Autodesk Inventor part; units mm, degrees
(part 2 of 2)
  spline S40 degree 3 poles (29.0897, 30.1625) (29.0266, 29.976) (28.9005, 29.603) (28.6866, 29.0523) (28.4534, 28.5096) (28.24, 28.066) (28.057, 27.7174) (27.9126, 27.4598) (27.7629, 27.2052) (27.6252, 27.0011) (27.525, 26.8315) (27.4755, 26.7183) (27.4493, 26.6233) (27.4363, 26.5506) (27.4305, 26.477) (27.4338, 26.403) (27.4493, 26.3306) (27.4734, 26.2607) (27.5066, 26.1943) (27.5982, 26.0779) (27.7581, 25.9243) (27.9005, 25.7542) (28.0104, 25.6549) (28.0744, 25.6173) (28.1424, 25.5885) (28.2136, 25.5681) (28.2872, 25.5597) (28.3611, 25.5605) (28.4345, 25.5685) (28.531, 25.5881) (28.6474, 25.6298) (28.8234, 25.7182) (29.0363, 25.8416) (29.3006, 25.9736) (29.5674, 26.1001) (29.9277, 26.2589) (30.3849, 26.4415) (30.9423, 26.6371) (31.5062, 26.8129) (31.8869, 26.9133) (32.0773, 26.9635) knots 0 0 0 0 0.059055 0.118109 0.177163 0.236216 0.265745 0.295273 0.3248 0.354329 0.36909 0.383846 0.391225 0.398597 0.405969 0.413352 0.420732 0.428104 0.435485 0.442861 0.472389 0.501917 0.509293 0.516674 0.524045 0.531426 0.538808 0.54618 0.553552 0.560931 0.575687 0.590449 0.619977 0.649505 0.679033 0.708561 0.767614 0.826668 0.885723 0.944777 0.944777 0.944777 0.944777
  spline S41 degree 3 poles (24.7117, 33.8426) (24.6746, 33.6492) (24.6004, 33.2625) (24.4634, 32.6879) (24.3064, 32.1185) (24.1553, 31.6499) (24.0215, 31.2796) (23.9135, 31.0048) (23.7999, 30.7321) (23.6913, 30.5112) (23.6151, 30.3296) (23.5814, 30.2107) (23.5685, 30.1131) (23.5655, 30.0393) (23.5698, 29.9655) (23.5831, 29.8926) (23.6083, 29.823) (23.6417, 29.7571) (23.6836, 29.6959) (23.7902, 29.593) (23.9695, 29.4625) (24.1338, 29.3135) (24.2562, 29.23) (24.3246, 29.2015) (24.396, 29.1822) (24.4693, 29.1717) (24.5433, 29.1734) (24.6164, 29.1842) (24.6881, 29.2022) (24.781, 29.2347) (24.8906, 29.2919) (25.0529, 29.4035) (25.2471, 29.5547) (25.491, 29.7214) (25.7381, 29.8831) (26.0734, 30.0894) (26.5014, 30.3327) (27.027, 30.6023) (27.5617, 30.8533) (27.9252, 31.0046) (28.107, 31.0803) knots 0 0 0 0 0.059055 0.118109 0.177163 0.236216 0.265745 0.295273 0.3248 0.354329 0.36909 0.383846 0.391225 0.398597 0.405969 0.413352 0.420732 0.428104 0.435485 0.442861 0.472389 0.501917 0.509293 0.516674 0.524045 0.531426 0.538808 0.54618 0.553552 0.560931 0.575687 0.590449 0.619977 0.649505 0.679033 0.708561 0.767614 0.826668 0.885723 0.944777 0.944777 0.944777 0.944777
  spline S42 degree 3 poles (19.8733, 36.8923) (19.8628, 36.6957) (19.842, 36.3025) (19.7846, 35.7145) (19.7065, 35.1291) (19.6207, 34.6443) (19.5385, 34.2592) (19.4689, 33.9723) (19.3935, 33.6866) (19.316, 33.453) (19.2653, 33.2627) (19.2481, 33.1403) (19.2486, 33.0418) (19.2556, 32.9683) (19.2699, 32.8958) (19.2931, 32.8255) (19.3275, 32.7599) (19.3696, 32.6991) (19.4194, 32.6442) (19.539, 32.5568) (19.7345, 32.452) (19.9175, 32.3267) (20.0501, 32.2607) (20.1218, 32.2417) (20.1951, 32.2323) (20.2692, 32.2319) (20.3423, 32.2437) (20.4132, 32.2643) (20.4818, 32.2919) (20.5694, 32.3368) (20.6702, 32.4084) (20.8158, 32.541) (20.9876, 32.7173) (21.2065, 32.9156) (21.4293, 33.1094) (21.7334, 33.3595) (22.1243, 33.6588) (22.6082, 33.9974) (23.1038, 34.3189) (23.4433, 34.5183) (23.6131, 34.618) knots 0 0 0 0 0.059055 0.118109 0.177163 0.236216 0.265745 0.295273 0.3248 0.354329 0.36909 0.383846 0.391225 0.398597 0.405969 0.413352 0.420732 0.428104 0.435485 0.442861 0.472389 0.501917 0.509293 0.516674 0.524045 0.531426 0.538808 0.54618 0.553552 0.560931 0.575687 0.590449 0.619977 0.649505 0.679033 0.708561 0.767614 0.826668 0.885723 0.944777 0.944777 0.944777 0.944777
  spline S43 degree 3 poles (14.6647, 39.2547) (14.6811, 39.0585) (14.714, 38.6662) (14.7372, 38.0759) (14.7395, 37.4852) (14.7205, 36.9933) (14.6916, 36.6006) (14.6617, 36.3069) (14.6259, 36.0136) (14.5809, 35.7716) (14.5566, 35.5762) (14.5562, 35.4526) (14.5701, 35.3551) (14.5871, 35.2832) (14.6111, 35.2134) (14.6436, 35.1468) (14.6867, 35.0865) (14.7366, 35.0321) (14.7935, 34.9844) (14.9239, 34.9141) (15.1318, 34.8369) (15.3301, 34.7377) (15.4705, 34.6904) (15.5442, 34.6813) (15.618, 34.682) (15.6915, 34.6916) (15.7623, 34.7133) (15.8298, 34.7434) (15.8939, 34.7801) (15.9747, 34.8365) (16.0647, 34.9211) (16.1909, 35.0723) (16.3371, 35.2703) (16.527, 35.4967) (16.7213, 35.719) (16.9885, 36.0082) (17.335, 36.3579) (17.7683, 36.7593) (18.2156, 37.1452) (18.5248, 37.389) (18.6793, 37.5109) knots 0 0 0 0 0.059055 0.118109 0.177163 0.236216 0.265745 0.295273 0.3248 0.354329 0.36909 0.383846 0.391225 0.398597 0.405969 0.413352 0.420732 0.428104 0.435485 0.442861 0.472389 0.501917 0.509293 0.516674 0.524045 0.531426 0.538808 0.54618 0.553552 0.560931 0.575687 0.590449 0.619977 0.649505 0.679033 0.708561 0.767614 0.826668 0.885723 0.944777 0.944777 0.944777 0.944777
  spline S44 degree 3 poles (9.1829, 40.8859) (9.2259, 40.6938) (9.3119, 40.3096) (9.4152, 39.728) (9.498, 39.1431) (9.5461, 38.6532) (9.571, 38.2602) (9.5814, 37.9651) (9.5858, 37.6698) (9.5742, 37.4239) (9.5767, 37.227) (9.5932, 37.1045) (9.6202, 37.0097) (9.6468, 36.9409) (9.6802, 36.8749) (9.7214, 36.8134) (9.7723, 36.7596) (9.8292, 36.7124) (9.892, 36.673) (10.0308, 36.6211) (10.2472, 36.5728) (10.4572, 36.5016) (10.6027, 36.4738) (10.6769, 36.4749) (10.75, 36.4856) (10.8215, 36.5052) (10.8887, 36.5363) (10.9514, 36.5753) (11.01, 36.6203) (11.0823, 36.6872) (11.16, 36.7833) (11.2645, 36.9503) (11.3823, 37.1664) (11.5396, 37.4165) (11.7018, 37.6632) (11.9272, 37.9861) (12.2229, 38.3797) (12.5975, 38.8363) (12.988, 39.2796) (13.2611, 39.5632) (13.3976, 39.705) knots 0 0 0 0 0.059055 0.118109 0.177163 0.236216 0.265745 0.295273 0.3248 0.354329 0.36909 0.383846 0.391225 0.398597 0.405969 0.413352 0.420732 0.428104 0.435485 0.442861 0.472389 0.501917 0.509293 0.516674 0.524045 0.531426 0.538808 0.54618 0.553552 0.560931 0.575687 0.590449 0.619977 0.649505 0.679033 0.708561 0.767614 0.826668 0.885723 0.944777 0.944777 0.944777 0.944777
  spline S45 degree 3 poles (3.5301, 41.7555) (3.5988, 41.5711) (3.7363, 41.2021) (3.9179, 40.64) (4.0796, 40.0719) (4.194, 39.593) (4.272, 39.2071) (4.3225, 38.9162) (4.3671, 38.6242) (4.3891, 38.379) (4.4184, 38.1842) (4.4514, 38.0651) (4.4911, 37.975) (4.5269, 37.9104) (4.5689, 37.8496) (4.6181, 37.7943) (4.6758, 37.7478) (4.7386, 37.7089) (4.8062, 37.6783) (4.9508, 37.6458) (5.1718, 37.6275) (5.3895, 37.5855) (5.5375, 37.5778) (5.6108, 37.589) (5.6818, 37.6096) (5.7499, 37.6387) (5.8123, 37.6787) (5.8691, 37.7259) (5.921, 37.7784) (5.9835, 37.8546) (6.0474, 37.9603) (6.1281, 38.14) (6.2155, 38.3701) (6.3372, 38.6393) (6.4643, 38.9058) (6.6436, 39.2563) (6.883, 39.6865) (7.1919, 40.19) (7.5184, 40.6823) (7.7504, 41.0004) (7.8664, 41.1595) knots 0 0 0 0 0.059055 0.118109 0.177163 0.236216 0.265745 0.295273 0.3248 0.354329 0.36909 0.383846 0.391225 0.398597 0.405969 0.413352 0.420732 0.428104 0.435485 0.442861 0.472389 0.501917 0.509293 0.516674 0.524045 0.531426 0.538808 0.54618 0.553552 0.560931 0.575687 0.590449 0.619977 0.649505 0.679033 0.708561 0.767614 0.826668 0.885723 0.944777 0.944777 0.944777 0.944777
  circle A4 centre (0, 0) radius 5
  circle A5 centre (0, 0) radius 10
  circle A6 centre (0, 0) radius 33
  line L0 (0, -58.6663) -> (0, 58.6663) construction
  line L1 (-5, 8.6603) -> (-5, 32.619)
  line L2 (5, 8.6603) -> (5, 32.619)
  line L3 (-8.6603, -5) -> (-32.619, -5)
  line L4 (-8.6603, 5) -> (-32.619, 5)
  line L5 (5, -8.6603) -> (5, -32.619)
  line L6 (-5, -8.6603) -> (-5, -32.619)
  line L7 (8.6603, 5) -> (32.619, 5)
  line L8 (8.6603, -5) -> (32.619, -5)
  point P0 (-1.9127, 41.3251)
  point P1 (-1.6555, 40.7935)
  point P2 (-1.4188, 40.2525)
  point P3 (-1.205, 39.702)
  point P4 (-1.1077, 39.4232)
  point P5 (-1.0178, 39.142)
  point P6 (-0.9358, 38.8583)
  point P7 (-0.8628, 38.5722)
  point P8 (-0.8193, 38.4311)
  point P9 (-0.7593, 38.2963)
  point P10 (-0.7207, 38.2334)
  point P11 (-0.6765, 38.1744)
  point P12 (-0.6265, 38.1203)
  point P13 (-0.57, 38.0727)
  point P14 (-0.507, 38.0343)
  point P15 (-0.4396, 38.0044)
  point P16 (-0.3686, 37.9843)
  point P17 (-0.2953, 37.9763)
  point P18 (0, 37.976)
  point P19 (0.2953, 37.9763)
  point P20 (0.3686, 37.9843)
  point P21 (0.4396, 38.0044)
  point P22 (0.507, 38.0343)
  point P23 (0.57, 38.0727)
  point P24 (0.6265, 38.1203)
  point P25 (0.6765, 38.1744)
  point P26 (0.7207, 38.2334)
  point P27 (0.7593, 38.2963)
  point P28 (0.8193, 38.4311)
  point P29 (0.8628, 38.5722)
  point P30 (0.9358, 38.8583)
  point P31 (1.0178, 39.142)
  point P32 (1.1077, 39.4232)
  point P33 (1.205, 39.702)
  point P34 (1.4188, 40.2525)
  point P35 (1.6555, 40.7935)
  point P36 (1.9127, 41.3251)
  point P37 (-7.522, 40.6798)
  point P38 (-7.1948, 40.1881)
  point P39 (-6.8866, 39.6844)
  point P40 (-6.5998, 39.1682)
  point P41 (-6.4656, 38.9052)
  point P42 (-6.3381, 38.6388)
  point P43 (-6.2183, 38.3689)
  point P44 (-6.1071, 38.0954)
  point P45 (-6.0447, 37.9616)
  point P46 (-5.9669, 37.8362)
  point P47 (-5.9201, 37.7792)
  point P48 (-5.8683, 37.7268)
  point P49 (-5.8114, 37.6799)
  point P50 (-4.3216, 38.916)
  point P51 (-5.7489, 37.6405)
  point P52 (-4.0755, 40.0708)
  point P53 (-3.7322, 41.2007)
  point P54 (-4.2124, 39.4963)
  point P55 (-4.2707, 39.2069)
  point P56 (-4.3641, 38.6238)
  point P57 (-4.3974, 38.3304)
  point P58 (-4.4214, 38.1847)
  point P59 (-4.4624, 38.043)
  point P60 (-4.4921, 37.9755)
  point P61 (-4.5279, 37.911)
  point P62 (-4.57, 37.8505)
  point P63 (-4.6195, 37.7957)
  point P64 (-4.6767, 37.7491)
  point P65 (-4.7394, 37.7103)
  point P66 (-4.807, 37.6807)
  point P67 (-4.8786, 37.6628)
  point P68 (-5.4636, 37.5824)
  point P69 (-5.5374, 37.5803)
  point P70 (-5.6105, 37.5906)
  point P71 (-5.6813, 37.611)
  point P72 (-5.1711, 37.6223)
  point P73 (-3.9146, 40.639)
  point P74 (-12.9912, 39.2766)
  point P75 (-12.6001, 38.8341)
  point P76 (-12.2262, 38.3771)
  point P77 (-11.8718, 37.9047)
  point P78 (-11.7029, 37.6624)
  point P79 (-11.5404, 37.4159)
  point P80 (-11.385, 37.1649)
  point P81 (-11.2375, 36.909)
  point P82 (-11.1575, 36.785)
  point P83 (-11.0634, 36.6713)
  point P84 (-11.0092, 36.6212)
  point P85 (-10.9507, 36.5763)
  point P86 (-10.888, 36.5376)
  point P87 (-9.5804, 37.9651)
  point P88 (-10.8208, 36.5071)
  point P89 (-9.4938, 39.1426)
  point P90 (-9.3076, 40.3087)
  point P91 (-9.5512, 38.5549)
  point P92 (-9.5696, 38.2602)
  point P93 (-9.5827, 37.6698)
  point P94 (-9.5758, 37.3746)
  point P95 (-9.5797, 37.227)
  point P96 (-9.6011, 37.081)
  point P97 (-9.6213, 37.0101)
  point P98 (-9.6479, 36.9414)
  point P99 (-9.6815, 36.8757)
  point P100 (-9.723, 36.8147)
  point P101 (-9.7733, 36.7607)
  point P102 (-9.8301, 36.7137)
  point P103 (-9.8931, 36.6752)
  point P104 (-9.9615, 36.6477)
  point P105 (-10.5302, 36.4883)
  point P106 (-10.603, 36.4763)
  point P107 (-10.6768, 36.4765)
  point P108 (-10.7497, 36.4871)
  point P109 (-10.2458, 36.5677)
  point P110 (-9.4118, 39.7274)
  point P111 (-18.2183, 37.1418)
  point P112 (-17.7707, 36.7567)
  point P113 (-17.338, 36.3548)
  point P114 (-16.9225, 35.9351)
  point P115 (-16.7223, 35.7181)
  point P116 (-16.5277, 35.496)
  point P117 (-16.3395, 35.2684)
  point P118 (-16.1586, 35.0351)
  point P119 (-16.0625, 34.9231)
  point P120 (-15.9537, 34.8233)
  point P121 (-15.8933, 34.781)
  point P122 (-15.8292, 34.7445)
  point P123 (-15.7618, 34.7147)
  point P124 (-14.6607, 36.3069)
  point P125 (-15.691, 34.6936)
  point P126 (-14.7353, 37.4853)
  point P127 (-14.7096, 38.6659)
  point P128 (-14.7121, 36.8952)
  point P129 (-14.6902, 36.6007)
  point P130 (-14.6229, 36.0141)
  point P131 (-14.5758, 35.7226)
  point P132 (-14.5595, 35.5759)
  point P133 (-14.5608, 35.4283)
  point P134 (-14.5712, 35.3553)
  point P135 (-14.5883, 35.2835)
  point P136 (-14.6125, 35.2139)
  point P137 (-14.6454, 35.1478)
  point P138 (-14.6879, 35.0875)
  point P139 (-14.7378, 35.0332)
  point P140 (-14.7949, 34.9865)
  point P141 (-14.859, 34.9499)
  point P142 (-15.4006, 34.7146)
  point P143 (-15.4711, 34.6928)
  point P144 (-15.5442, 34.6829)
  point P145 (-15.6179, 34.6835)
  point P146 (-15.1297, 34.832)
  point P147 (-14.7337, 38.0758)
  point P148 (-23.1061, 34.3152)
  point P149 (-22.6102, 33.9946)
  point P150 (-22.1268, 33.6554)
  point P151 (-21.6581, 33.2961)
  point P152 (-21.4302, 33.1084)
  point P153 (-21.2071, 32.9149)
  point P154 (-20.9897, 32.7151)
  point P155 (-20.7787, 32.5085)
  point P156 (-20.6682, 32.4106)
  point P157 (-20.5469, 32.3266)
  point P158 (-20.4813, 32.2929)
  point P159 (-20.4128, 32.2655)
  point P160 (-20.342, 32.2452)
  point P161 (-19.468, 33.9725)
  point P162 (-20.269, 32.2339)
  point P163 (-19.7023, 35.1297)
  point P164 (-19.8376, 36.3028)
  point P165 (-19.599, 34.5483)
  point P166 (-19.5372, 34.2595)
  point P167 (-19.3906, 33.6875)
  point P168 (-19.3043, 33.4051)
  point P169 (-19.2682, 33.262)
  point P170 (-19.2494, 33.1156)
  point P171 (-19.2497, 33.0419)
  point P172 (-19.2568, 32.9685)
  point P173 (-19.2714, 32.8962)
  point P174 (-19.295, 32.8263)
  point P175 (-19.3288, 32.7607)
  point P176 (-19.3709, 32.7001)
  point P177 (-19.4211, 32.6461)
  point P178 (-19.4796, 32.6011)
  point P179 (-19.9842, 32.2942)
  point P180 (-20.051, 32.263)
  point P181 (-20.1221, 32.2433)
  point P182 (-20.1952, 32.2338)
  point P183 (-19.7317, 32.4474)
  point P184 (-19.7811, 35.715)
  point P185 (-27.5635, 30.8493)
  point P186 (-27.0285, 30.5992)
  point P187 (-26.5034, 30.329)
  point P188 (-25.9902, 30.0369)
  point P189 (-25.7388, 29.882)
  point P190 (-25.4915, 29.7206)
  point P191 (-25.2489, 29.5522)
  point P192 (-25.0118, 29.3763)
  point P193 (-24.889, 29.2944)
  point P194 (-24.7574, 29.2277)
  point P195 (-24.6877, 29.2033)
  point P196 (-24.6162, 29.1854)
  point P197 (-24.5432, 29.1749)
  point P198 (-23.9125, 31.0052)
  point P199 (-24.4694, 29.1737)
  dimension "d4" = 360
  dimension "d6" = 10
  dimension "d7" = 20
  dimension "d8" = 66
  dimension "d9" = 5
  dimension "d10" = 5
  dimension "d13" = 360
  constraints: 16 end point, 6 centre point, 4 point on circle, 3 coincident, 2 vertical, 3706 other
  measures "d6" diameter of A4
  measures "d7" diameter of A5
  measures "d8" diameter of A6
  measures "d9" distance between parallel lines of L0 L1
  measures "d10" distance between parallel lines of L2 L0
extrude "Выдавливание1" add sketch "Sketch1" against normal blind 6 contours S0 A3 S45 S44 S43 S42 S41 S40 S39 S38 S37 S36 S35 S34 S33 S32 S31 S30 S29 S28 S27 S26 S25 S24 S23 S22 S21 S20 S19 S18 S17 S16 S15 S14 S13 S12 S11 S10 S9 S8 S7 S6 S5 S4 S3 S2 S1 | A5 | A5 L7 A6 L8 | A5 L1 A6 L2 | L5 A6 L6 A5 | A5 L3 A6 L4
fillet "Сопряжение1" radius 5 16 edges at (-8.6603, -5, -3) (-5, -8.6603, -3) (-32.619, -5, -3) (-5, -32.619, -3) (5, -8.6603, -3) (8.6603, -5, -3) (5, -32.619, -3) (32.619, -5, -3) (-5, 8.6603, -3) (-8.6603, 5, -3) (-5, 32.619, -3) (-32.619, 5, -3) (5, 8.6603, -3) (5, 32.619, -3) (8.6603, 5, -3) (32.619, 5, -3)
equation "\"d0\" = Ширина_грани"
equation "\"Модуль\" = 1.746"
equation "\"Угол_зацепления\" = 20deg"
equation "\"Зазор_профиля_зуба\" = 0.25"
equation "\"Радиус_закругления_зуба\" = 0.2386"
equation "\"Диаметр_головки\" = 83.80895"
equation "\"Диаметр_впадин\" = 75.95195"
equation "\"Основной_диаметр\" = 75.47235"
equation "\"Средний_диаметр\" = 80.316"
equation "\"Ширина_грани\" = 6"
equation "\"Коэффициент_смещения\" = 0.000272"
equation "\"Изменение_высоты_головки_зуба\" = 0"
equation "\"Окружной_шаг\" = 5.48522"
equation "\"Общий_сдвиг_инструмента\" = 0.00048"
equation "\"Внутренний\" = 0"
